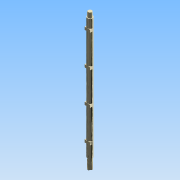
# Autodesk Inventor part: 刀轴
Saved by Autodesk Inventor 2015 (Build 190159000, 159)
## iProperties
Created: 2017-05-18
Part Number: 刀轴
Material: 常规
Document SubType Name: Modeling
Designer: Administrator
Density: 1 g/cm^3
Appearance: 镍
Author: Administrator
Autodesk Inventor part; units mm, degrees
ref_plane "YZ Plane" through (0, 0, 0) normal (1, 0, 0) x (0, 1, 0)
ref_plane "XZ Plane" through (0, 0, 0) normal (0, 1, 0) x (-1, 0, 0)
sketch "草图1" plane through (0, 0, 0) normal (0, 0, 1) x (1, 0, 0)
  circle A0 centre (0, 0) radius 10
  dimension "d0" = 20
  constraints: 1 centre point, 1 coincident
  measures "d0" diameter of A0
extrude "拉伸1" add sketch "草图1" along normal blind 447
sketch "草图2" plane through (0, 0, 447) normal (0, 0, 1) x (1, 0, 0)
  circle A0 centre (0, 0) radius 7.5
  dimension "d3" = 15
  constraints: 1 centre point, 1 coincident
  measures "d3" diameter of A0
extrude "拉伸2" add sketch "草图2" along normal blind 18
chamfer "倒角1" distance 1 angle 45 1 edges at (-7.5, 0, 465)
sketch "草图3" plane through (0, 0, 0) normal (0, 0, -1) x (-1, 0, 0)
  circle A0 centre (0, 0) radius 7.5
  dimension "d9" = 15
  constraints: 1 centre point, 1 coincident
  measures "d9" diameter of A0
extrude "拉伸3" add sketch "草图3" along normal blind 40
ref_plane "工作平面1" through (0, 0, 45) normal (0, 0, -1) x (-1, 0, 0)
sketch "草图4" plane through (0, 0, 45) normal (0, 0, -1) x (-1, 0, 0)
  circle A0 centre (0, 0) radius 10
  circle A1 centre (0, 0) radius 10 projected
  line L0 (0, 10) -> (10, 10)
  line L1 (10, 0) -> (10, -10)
  line L2 (10, -10) -> (-10, -10)
  line L3 (-10, -10) -> (-10, 0)
  dimension "d13" = 20
  dimension "d14" = 20
  dimension "d15" = 10
  dimension "d16" = 10
  constraints: 8 end point, 3 point on circle, 2 parallel, 2 tangent, 1 centre point, 1 concentric, 1 horizontal, 1 perpendicular
  measures "d13" diameter of A0
  measures "d14" distance of L1.end L2.end
  measures "d15" distance of L0.start L0.end
  measures "d16" horizontal distance of point (0, 0) L0.end
extrude "拉伸4" add sketch "草图4" against normal blind 10 contours L1 L2 A0 | L2 L3 A0
pattern_linear "矩形阵列1" count 4 spacing 120 along (0, 0, 1) of "拉伸4"
sketch "草图5" plane through (0, 0, -40) normal (0, 0, -1) x (-1, 0, 0)
  circle A0 centre (0, 0) radius 7.5
  line L0 (7.2712, -1.8385) -> (1.0192, 7.4304)
  line L1 (-1.0192, -7.4304) -> (-7.2712, 1.8385)
  line L2 (-10, -10) -> (0, -10) projected
  dimension "d22" = 15
  dimension "d23" = 10
  dimension "d24" = 56
  constraints: 4 end point, 4 point on circle, 2 parallel, 1 centre point, 1 coincident
  measures "d22" diameter of A0
  measures "d23" distance between parallel lines of L1 L0
  measures "d24" angle of L2 L1
extrude "拉伸5" cut sketch "草图5" against normal blind 20 contours A0 L0 | L1 A0
